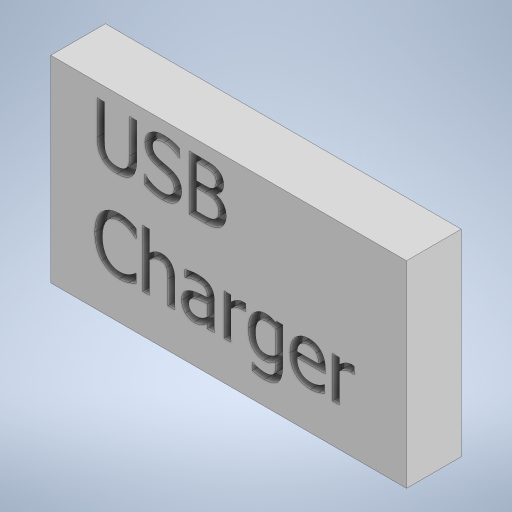
# Autodesk Inventor part: rapoukUSBChargerv0
Saved by Autodesk Inventor 2024 (Build 280153000, 153)
## iProperties
Created: 2024-02-03
Part Number: rapoukUSBChargerv0
Material: Všeobecné
Document SubType Name: Modeling
Designer: Roman Suk
Density: 1 g/cm^3
Appearance: Výchozí
Author: Roman Suk
MASSSFP: 400 g
SFP: 4HR
Autodesk Inventor part; units mm, degrees
ref_plane "YZ Plane" through (0, 0, 0) normal (1, 0, 0) x (0, 1, 0)
ref_plane "XZ Plane" through (0, 0, 0) normal (0, 1, 0) x (-1, 0, 0)
ref_plane "XY Plane" through (0, 0, 0) normal (0, 0, 1) x (1, 0, 0)
sketch "Sketch2" plane through (0, 0, 0) normal (0, 0, 1) x (1, 0, 0)
  line L0 (-16.25, -9) -> (16.25, -9)
  line L1 (16.25, -9) -> (16.25, 9)
  line L2 (16.25, 9) -> (-16.25, 9)
  line L3 (-16.25, 9) -> (-16.25, -9)
  line L4 (-16.25, -9) -> (16.25, 9) construction
  line L5 (16.25, -9) -> (-16.25, 9) construction
  point P0 (0, 0)
  dimension "d2" = 32.5
  dimension "d3" = 18
  constraints: 12 end point, 2 midpoint, 2 parallel, 1 horizontal, 1 perpendicular
  measures "d2" distance of L2.end L1.end
  measures "d3" distance of L1.end L0.end
extrude "Extrusion2" add sketch "Sketch2" along normal blind 5
sketch "Sketch3" plane through (0, 0, 5) normal (0, 0, 1) x (1, 0, 0)
  line L0 (-12.4484, 7.8564) -> (20.0688, 7.8564) construction
  line L1 (20.0688, 7.8564) -> (20.0688, -10.2359) construction
  line L2 (20.0688, -10.2359) -> (-12.4484, -10.2359) construction
  line L3 (-12.4484, -10.2359) -> (-12.4484, 7.8564) construction
  spline S0 degree 2 poles (-10.1956, 2.662) (-10.6373, 2.662) (-11.2937, 2.8929) (-11.5246, 3.1239) knots 0 0 0 1 2 2 2
  spline S1 degree 2 poles (-11.5246, 3.1239) (-11.788, 3.3832) (-12.0027, 4.1125) (-12.0027, 4.6474) knots 0 0 0 1 2 2 2
  line L4 (-12.0027, 4.6474) -> (-12.0027, 7.7673)
  line L5 (-12.0027, 7.7673) -> (-11.3382, 7.7673)
  line L6 (-11.3382, 7.7673) -> (-11.3382, 4.6474)
  spline S2 degree 2 poles (-11.3382, 4.6474) (-11.3382, 4.2989) (-11.2491, 3.8289) (-11.1235, 3.6385) knots 0 0 0 1 2 2 2
  spline S3 degree 2 poles (-11.1235, 3.6385) (-10.9898, 3.4359) (-10.5279, 3.2292) (-10.1956, 3.2292) knots 0 0 0 1 2 2 2
  spline S4 degree 2 poles (-10.1956, 3.2292) (-9.8836, 3.2292) (-9.3974, 3.4359) (-9.2637, 3.6385) knots 0 0 0 1 2 2 2
  spline S5 degree 2 poles (-9.2637, 3.6385) (-9.1381, 3.8289) (-9.0489, 4.2949) (-9.0489, 4.6312) knots 0 0 0 1 2 2 2
  line L7 (-9.0489, 4.6312) -> (-9.0489, 7.7673)
  line L8 (-9.0489, 7.7673) -> (-8.3844, 7.7673)
  line L9 (-8.3844, 7.7673) -> (-8.3844, 4.6474)
  spline S6 degree 2 poles (-8.3844, 4.6474) (-8.3844, 4.1247) (-8.5951, 3.3791) (-8.8625, 3.1239) knots 0 0 0 1 2 2 2
  spline S7 degree 2 poles (-8.8625, 3.1239) (-9.1016, 2.8889) (-9.7337, 2.662) (-10.1956, 2.662) knots 0 0 0 1 2 2 2
  spline S8 degree 2 poles (-6.0384, 2.6782) (-6.5813, 2.6782) (-7.3431, 2.9051) (-7.6794, 3.0671) knots 0 0 0 1 2 2 2
  line L10 (-7.6794, 3.0671) -> (-7.6794, 3.9018)
  line L11 (-7.6794, 3.9018) -> (-7.6308, 3.9018)
  spline S9 degree 2 poles (-7.6308, 3.9018) (-7.3026, 3.5939) (-6.4719, 3.2535) (-6.087, 3.2535) knots 0 0 0 1 2 2 2
  spline S10 degree 2 poles (-6.087, 3.2535) (-5.536, 3.2535) (-4.9727, 3.7114) (-4.9727, 4.0882) knots 0 0 0 1 2 2 2
  spline S11 degree 2 poles (-4.9727, 4.0882) (-4.9727, 4.388) (-5.2685, 4.7608) (-5.5886, 4.854) knots 0 0 0 1 2 2 2
  spline S12 degree 2 poles (-5.5886, 4.854) (-5.8196, 4.9188) (-6.2045, 5.008) (-6.4922, 5.0809) knots 0 0 0 1 2 2 2
  spline S13 degree 2 poles (-6.4922, 5.0809) (-6.7515, 5.1498) (-7.1608, 5.3564) (-7.3188, 5.5226) knots 0 0 0 1 2 2 2
  spline S14 degree 2 poles (-7.3188, 5.5226) (-7.4727, 5.6887) (-7.6429, 6.1344) (-7.6429, 6.4261) knots 0 0 0 1 2 2 2
  spline S15 degree 2 poles (-7.6429, 6.4261) (-7.6429, 7.0339) (-6.6948, 7.8564) (-5.9614, 7.8564) knots 0 0 0 1 2 2 2
  spline S16 degree 2 poles (-5.9614, 7.8564) (-5.54, 7.8564) (-4.7945, 7.6903) (-4.4744, 7.5323) knots 0 0 0 1 2 2 2
  line L12 (-4.4744, 7.5323) -> (-4.4744, 6.7381)
  line L13 (-4.4744, 6.7381) -> (-4.523, 6.7381)
  spline S17 degree 2 poles (-4.523, 6.7381) (-4.762, 6.9569) (-5.5076, 7.2811) (-5.9168, 7.2811) knots 0 0 0 1 2 2 2
  spline S18 degree 2 poles (-5.9168, 7.2811) (-6.3787, 7.2811) (-6.9501, 6.8475) (-6.9501, 6.495) knots 0 0 0 1 2 2 2
  spline S19 degree 2 poles (-6.9501, 6.495) (-6.9501, 6.179) (-6.6138, 5.8021) (-6.2977, 5.7171) knots 0 0 0 1 2 2 2
  spline S20 degree 2 poles (-6.2977, 5.7171) (-6.087, 5.6603) (-5.4752, 5.5145) (-5.2726, 5.4537) knots 0 0 0 1 2 2 2
  spline S21 degree 2 poles (-5.2726, 5.4537) (-4.758, 5.2957) (-4.2799, 4.6595) (-4.2799, 4.1936) knots 0 0 0 1 2 2 2
  spline S22 degree 2 poles (-4.2799, 4.1936) (-4.2799, 3.8978) (-4.5189, 3.3305) (-4.7337, 3.132) knots 0 0 0 1 2 2 2
  spline S23 degree 2 poles (-4.7337, 3.132) (-4.9727, 2.9132) (-5.5805, 2.6782) (-6.0384, 2.6782) knots 0 0 0 1 2 2 2
  spline S24 degree 2 poles (-0.2118, 4.303) (-0.2118, 3.9302) (-0.4954, 3.3589) (-0.7304, 3.1725) knots 0 0 0 1 2 2 2
  spline S25 degree 2 poles (-0.7304, 3.1725) (-1.0141, 2.9537) (-1.6583, 2.7673) (-2.1689, 2.7673) knots 0 0 0 1 2 2 2
  line L14 (-2.1689, 2.7673) -> (-3.6032, 2.7673)
  line L15 (-3.6032, 2.7673) -> (-3.6032, 7.7673)
  line L16 (-3.6032, 7.7673) -> (-2.2783, 7.7673)
  spline S26 degree 2 poles (-2.2783, 7.7673) (-1.7434, 7.7673) (-1.2086, 7.6984) (-0.9655, 7.5647) knots 0 0 0 1 2 2 2
  spline S27 degree 2 poles (-0.9655, 7.5647) (-0.694, 7.4229) (-0.4468, 6.9569) (-0.4468, 6.6409) knots 0 0 0 1 2 2 2
  spline S28 degree 2 poles (-0.4468, 6.6409) (-0.4468, 6.2884) (-0.8196, 5.7292) (-1.1478, 5.5712) knots 0 0 0 1 2 2 2
  line L17 (-1.1478, 5.5712) -> (-1.1478, 5.5469)
  spline S29 degree 2 poles (-1.1478, 5.5469) (-0.7021, 5.4253) (-0.2118, 4.7811) (-0.2118, 4.303) knots 0 0 0 1 2 2 2
  spline S30 degree 2 poles (-0.9047, 4.2746) (-0.9047, 4.5582) (-1.0667, 4.9229) (-1.3099, 5.0526) knots 0 0 0 1 2 2 2
  spline S31 degree 2 poles (-1.3099, 5.0526) (-1.4679, 5.1336) (-1.8407, 5.1822) (-2.1851, 5.1822) knots 0 0 0 1 2 2 2
  line L18 (-2.1851, 5.1822) -> (-2.9387, 5.1822)
  line L19 (-2.9387, 5.1822) -> (-2.9387, 3.3346)
  line L20 (-2.9387, 3.3346) -> (-2.3998, 3.3346)
  spline S32 degree 2 poles (-2.3998, 3.3346) (-1.9622, 3.3346) (-1.4598, 3.4156) (-1.2653, 3.5453) knots 0 0 0 1 2 2 2
  spline S33 degree 2 poles (-1.2653, 3.5453) (-1.0789, 3.679) (-0.9047, 4.0112) (-0.9047, 4.2746) knots 0 0 0 1 2 2 2
  spline S34 degree 2 poles (-1.1397, 6.5477) (-1.1397, 6.726) (-1.2612, 6.9934) (-1.395, 7.0704) knots 0 0 0 1 2 2 2
  spline S35 degree 2 poles (-1.395, 7.0704) (-1.557, 7.1595) (-1.9501, 7.2) (-2.3026, 7.2) knots 0 0 0 1 2 2 2
  line L21 (-2.3026, 7.2) -> (-2.9387, 7.2)
  line L22 (-2.9387, 7.2) -> (-2.9387, 5.7373)
  line L23 (-2.9387, 5.7373) -> (-2.1851, 5.7373)
  spline S36 degree 2 poles (-2.1851, 5.7373) (-1.8731, 5.7373) (-1.5773, 5.8021) (-1.4193, 5.9034) knots 0 0 0 1 2 2 2
  spline S37 degree 2 poles (-1.4193, 5.9034) (-1.2653, 6.0007) (-1.1397, 6.3127) (-1.1397, 6.5477) knots 0 0 0 1 2 2 2
  spline S38 degree 2 poles (-9.989, -5.5542) (-10.4752, -5.5542) (-11.2977, -5.226) (-11.5975, -4.8978) knots 0 0 0 1 2 2 2
  spline S39 degree 2 poles (-11.5975, -4.8978) (-11.8974, -4.5737) (-12.2256, -3.6012) (-12.2256, -2.9691) knots 0 0 0 1 2 2 2
  spline S40 degree 2 poles (-12.2256, -2.9691) (-12.2256, -2.3411) (-11.9055, -1.4092) (-11.6016, -1.0647) knots 0 0 0 1 2 2 2
  spline S41 degree 2 poles (-11.6016, -1.0647) (-11.3018, -0.7284) (-10.4833, -0.3759) (-9.9768, -0.3759) knots 0 0 0 1 2 2 2
  spline S42 degree 2 poles (-9.9768, -0.3759) (-9.7256, -0.3759) (-9.2839, -0.4489) (-9.0975, -0.5056) knots 0 0 0 1 2 2 2
  spline S43 degree 2 poles (-9.0975, -0.5056) (-8.9355, -0.5583) (-8.5992, -0.7082) (-8.433, -0.7973) knots 0 0 0 1 2 2 2
  line L24 (-8.433, -0.7973) -> (-8.433, -1.5996)
  line L25 (-8.433, -1.5996) -> (-8.4857, -1.5996)
  spline S44 degree 2 poles (-8.4857, -1.5996) (-8.5749, -1.5186) (-8.8504, -1.2916) (-9.0489, -1.1822) knots 0 0 0 1 2 2 2
  spline S45 degree 2 poles (-9.0489, -1.1822) (-9.2394, -1.0769) (-9.6891, -0.9432) (-9.9808, -0.9432) knots 0 0 0 1 2 2 2
  spline S46 degree 2 poles (-9.9808, -0.9432) (-10.3009, -0.9432) (-10.8723, -1.2066) (-11.087, -1.4578) knots 0 0 0 1 2 2 2
  spline S47 degree 2 poles (-11.087, -1.4578) (-11.2977, -1.713) (-11.5327, -2.4869) (-11.5327, -2.9691) knots 0 0 0 1 2 2 2
  spline S48 degree 2 poles (-11.5327, -2.9691) (-11.5327, -3.4837) (-11.2856, -4.2252) (-11.0708, -4.4805) knots 0 0 0 1 2 2 2
  spline S49 degree 2 poles (-11.0708, -4.4805) (-10.8601, -4.7276) (-10.2969, -4.9788) (-9.9808, -4.9788) knots 0 0 0 1 2 2 2
  spline S50 degree 2 poles (-9.9808, -4.9788) (-9.6932, -4.9788) (-9.2029, -4.837) (-9.0125, -4.7317) knots 0 0 0 1 2 2 2
  spline S51 degree 2 poles (-9.0125, -4.7317) (-8.8301, -4.6263) (-8.5586, -4.4075) (-8.4817, -4.3305) knots 0 0 0 1 2 2 2
  line L26 (-8.4817, -4.3305) -> (-8.433, -4.3305)
  line L27 (-8.433, -4.3305) -> (-8.433, -5.1247)
  spline S52 degree 2 poles (-8.433, -5.1247) (-8.5992, -5.2017) (-8.8909, -5.3435) (-9.0975, -5.4083) knots 0 0 0 1 2 2 2
  spline S53 degree 2 poles (-9.0975, -5.4083) (-9.3163, -5.4813) (-9.6891, -5.5542) (-9.989, -5.5542) knots 0 0 0 1 2 2 2
  line L28 (-4.916, -5.4651) -> (-5.5481, -5.4651)
  line L29 (-5.5481, -5.4651) -> (-5.5481, -3.3257)
  spline S54 degree 2 poles (-5.5481, -3.3257) (-5.5481, -3.0664) (-5.5967, -2.6207) (-5.6697, -2.4869) knots 0 0 0 1 2 2 2
  spline S55 degree 2 poles (-5.6697, -2.4869) (-5.7467, -2.3451) (-6.0222, -2.2074) (-6.2572, -2.2074) knots 0 0 0 1 2 2 2
  spline S56 degree 2 poles (-6.2572, -2.2074) (-6.4922, -2.2074) (-6.9906, -2.4586) (-7.2296, -2.6612) knots 0 0 0 1 2 2 2
  line L30 (-7.2296, -2.6612) -> (-7.2296, -5.4651)
  line L31 (-7.2296, -5.4651) -> (-7.8617, -5.4651)
  line L32 (-7.8617, -5.4651) -> (-7.8617, -0.2422)
  line L33 (-7.8617, -0.2422) -> (-7.2296, -0.2422)
  line L34 (-7.2296, -0.2422) -> (-7.2296, -2.1304)
  spline S57 degree 2 poles (-7.2296, -2.1304) (-6.946, -1.8751) (-6.399, -1.6077) (-6.0911, -1.6077) knots 0 0 0 1 2 2 2
  spline S58 degree 2 poles (-6.0911, -1.6077) (-5.54, -1.6077) (-4.916, -2.337) (-4.916, -3.0299) knots 0 0 0 1 2 2 2
  line L35 (-4.916, -3.0299) -> (-4.916, -5.4651)
  spline S59 degree 2 poles (-1.9379, -5.068) (-2.0149, -5.1247) (-2.2742, -5.3273) (-2.3958, -5.3881) knots 0 0 0 1 2 2 2
  spline S60 degree 2 poles (-2.3958, -5.3881) (-2.5619, -5.4772) (-2.8739, -5.5704) (-3.1575, -5.5704) knots 0 0 0 1 2 2 2
  spline S61 degree 2 poles (-3.1575, -5.5704) (-3.3885, -5.5704) (-3.8058, -5.3962) (-3.9638, -5.2382) knots 0 0 0 1 2 2 2
  spline S62 degree 2 poles (-3.9638, -5.2382) (-4.1138, -5.0842) (-4.2961, -4.6304) (-4.2961, -4.3792) knots 0 0 0 1 2 2 2
  spline S63 degree 2 poles (-4.2961, -4.3792) (-4.2961, -3.9902) (-3.9679, -3.4391) (-3.6113, -3.2811) knots 0 0 0 1 2 2 2
  spline S64 degree 2 poles (-3.6113, -3.2811) (-3.2953, -3.1352) (-2.4363, -3.0258) (-1.9379, -2.9975) knots 0 0 0 1 2 2 2
  line L36 (-1.9379, -2.9975) -> (-1.9379, -2.8759)
  spline S65 degree 2 poles (-1.9379, -2.8759) (-1.9379, -2.6571) (-2.0716, -2.3856) (-2.1932, -2.3087) knots 0 0 0 1 2 2 2
  spline S66 degree 2 poles (-2.1932, -2.3087) (-2.3147, -2.2317) (-2.6632, -2.1831) (-2.8496, -2.1831) knots 0 0 0 1 2 2 2
  spline S67 degree 2 poles (-2.8496, -2.1831) (-3.0684, -2.1831) (-3.6599, -2.3127) (-3.9557, -2.4383) knots 0 0 0 1 2 2 2
  line L37 (-3.9557, -2.4383) -> (-3.9922, -2.4383)
  line L38 (-3.9922, -2.4383) -> (-3.9922, -1.7941)
  spline S68 degree 2 poles (-3.9922, -1.7941) (-3.818, -1.7455) (-3.1656, -1.6239) (-2.8455, -1.6239) knots 0 0 0 1 2 2 2
  spline S69 degree 2 poles (-2.8455, -1.6239) (-2.4565, -1.6239) (-1.9257, -1.7455) (-1.715, -1.9035) knots 0 0 0 1 2 2 2
  spline S70 degree 2 poles (-1.715, -1.9035) (-1.5084, -2.0574) (-1.3058, -2.5477) (-1.3058, -2.9002) knots 0 0 0 1 2 2 2
  line L39 (-1.3058, -2.9002) -> (-1.3058, -5.4651)
  line L40 (-1.3058, -5.4651) -> (-1.9379, -5.4651)
  line L41 (-1.9379, -5.4651) -> (-1.9379, -5.068)
  line L42 (-1.9379, -4.5412) -> (-1.9379, -3.4999)
  spline S71 degree 2 poles (-1.9379, -3.4999) (-2.1648, -3.5202) (-2.8496, -3.5891) (-3.0643, -3.6539) knots 0 0 0 1 2 2 2
  spline S72 degree 2 poles (-3.0643, -3.6539) (-3.3155, -3.7309) (-3.6437, -4.051) (-3.6437, -4.3346) knots 0 0 0 1 2 2 2
  spline S73 degree 2 poles (-3.6437, -4.3346) (-3.6437, -4.6587) (-3.2791, -4.9869) (-2.9306, -4.9869) knots 0 0 0 1 2 2 2
  spline S74 degree 2 poles (-2.9306, -4.9869) (-2.6348, -4.9869) (-2.1486, -4.7317) (-1.9379, -4.5412) knots 0 0 0 1 2 2 2
  line L43 (1.571, -2.3897) -> (1.5386, -2.3897)
  spline S75 degree 2 poles (1.5386, -2.3897) (1.4657, -2.3694) (1.3076, -2.3613) (1.1982, -2.3613) knots 0 0 0 1 2 2 2
  spline S76 degree 2 poles (1.1982, -2.3613) (0.943, -2.3613) (0.4405, -2.5842) (0.2136, -2.803) knots 0 0 0 1 2 2 2
  line L44 (0.2136, -2.803) -> (0.2136, -5.4651)
  line L45 (0.2136, -5.4651) -> (-0.4185, -5.4651)
  line L46 (-0.4185, -5.4651) -> (-0.4185, -1.713)
  line L47 (-0.4185, -1.713) -> (0.2136, -1.713)
  line L48 (0.2136, -1.713) -> (0.2136, -2.2722)
  spline S77 degree 2 poles (0.2136, -2.2722) (0.558, -1.9643) (1.0726, -1.713) (1.3157, -1.713) knots 0 0 0 1 2 2 2
  spline S78 degree 2 poles (1.3157, -1.713) (1.413, -1.713) (1.5102, -1.7211) (1.571, -1.7333) knots 0 0 0 1 2 2 2
  line L49 (1.571, -1.7333) -> (1.571, -2.3897)
  spline S79 degree 2 poles (2.195, -6.0647) (2.2598, -6.0931) (2.507, -6.1822) (2.665, -6.2187) knots 0 0 0 1 2 2 2
  spline S80 degree 2 poles (2.665, -6.2187) (2.8392, -6.2633) (3.135, -6.316) (3.3093, -6.316) knots 0 0 0 1 2 2 2
  spline S81 degree 2 poles (3.3093, -6.316) (3.601, -6.316) (4.0062, -6.162) (4.1196, -6.0242) knots 0 0 0 1 2 2 2
  spline S82 degree 2 poles (4.1196, -6.0242) (4.229, -5.8865) (4.3141, -5.5258) (4.3141, -5.2949) knots 0 0 0 1 2 2 2
  line L50 (4.3141, -5.2949) -> (4.3141, -4.9667)
  spline S83 degree 2 poles (4.3141, -4.9667) (4.0589, -5.1895) (3.5686, -5.4002) (3.1999, -5.4002) knots 0 0 0 1 2 2 2
  spline S84 degree 2 poles (3.1999, -5.4002) (2.5597, -5.4002) (1.802, -4.448) (1.802, -3.5526) knots 0 0 0 1 2 2 2
  spline S85 degree 2 poles (1.802, -3.5526) (1.802, -3.0866) (2.0653, -2.3654) (2.2841, -2.1101) knots 0 0 0 1 2 2 2
  spline S86 degree 2 poles (2.2841, -2.1101) (2.4948, -1.8711) (3.0743, -1.6077) (3.3822, -1.6077) knots 0 0 0 1 2 2 2
  spline S87 degree 2 poles (3.3822, -1.6077) (3.6739, -1.6077) (4.0994, -1.7455) (4.3141, -1.8711) knots 0 0 0 1 2 2 2
  line L51 (4.3141, -1.8711) -> (4.3506, -1.713)
  line L52 (4.3506, -1.713) -> (4.9462, -1.713)
  line L53 (4.9462, -1.713) -> (4.9462, -5.0356)
  spline S88 degree 2 poles (4.9462, -5.0356) (4.9462, -5.9918) (4.1156, -6.8832) (3.2606, -6.8832) knots 0 0 0 1 2 2 2
  spline S89 degree 2 poles (3.2606, -6.8832) (2.9851, -6.8832) (2.4097, -6.7941) (2.1626, -6.7211) knots 0 0 0 1 2 2 2
  line L54 (2.1626, -6.7211) -> (2.1626, -6.0647)
  line L55 (2.1626, -6.0647) -> (2.195, -6.0647)
  line L56 (4.3141, -4.448) -> (4.3141, -2.3856)
  spline S90 degree 2 poles (4.3141, -2.3856) (4.0791, -2.2722) (3.682, -2.175) (3.4835, -2.175) knots 0 0 0 1 2 2 2
  spline S91 degree 2 poles (3.4835, -2.175) (3.0054, -2.175) (2.4543, -2.88) (2.4543, -3.5404) knots 0 0 0 1 2 2 2
  spline S92 degree 2 poles (2.4543, -3.5404) (2.4543, -4.1644) (2.8717, -4.8168) (3.3417, -4.8168) knots 0 0 0 1 2 2 2
  spline S93 degree 2 poles (3.3417, -4.8168) (3.5888, -4.8168) (4.1075, -4.6223) (4.3141, -4.448) knots 0 0 0 1 2 2 2
  spline S94 degree 2 poles (7.4908, -5.5502) (6.5913, -5.5502) (5.6026, -4.5412) (5.6026, -3.6093) knots 0 0 0 1 2 2 2
  spline S95 degree 2 poles (5.6026, -3.6093) (5.6026, -2.6936) (6.5629, -1.6077) (7.3368, -1.6077) knots 0 0 0 1 2 2 2
  spline S96 degree 2 poles (7.3368, -1.6077) (7.6853, -1.6077) (8.2242, -1.8103) (8.4227, -2.025) knots 0 0 0 1 2 2 2
  spline S97 degree 2 poles (8.4227, -2.025) (8.6253, -2.2398) (8.8401, -2.8597) (8.8401, -3.3095) knots 0 0 0 1 2 2 2
  line L57 (8.8401, -3.3095) -> (8.8401, -3.6539)
  line L58 (8.8401, -3.6539) -> (6.2428, -3.6539)
  spline S98 degree 2 poles (6.2428, -3.6539) (6.2428, -4.3062) (6.8992, -4.9991) (7.4827, -4.9991) knots 0 0 0 1 2 2 2
  spline S99 degree 2 poles (7.4827, -4.9991) (7.6893, -4.9991) (8.0905, -4.9059) (8.2525, -4.833) knots 0 0 0 1 2 2 2
  spline S100 degree 2 poles (8.2525, -4.833) (8.4227, -4.7519) (8.6577, -4.6101) (8.7347, -4.5453) knots 0 0 0 1 2 2 2
  line L59 (8.7347, -4.5453) -> (8.7712, -4.5453)
  line L60 (8.7712, -4.5453) -> (8.7712, -5.2341)
  spline S101 degree 2 poles (8.7712, -5.2341) (8.6618, -5.2787) (8.3295, -5.4083) (8.1999, -5.4448) knots 0 0 0 1 2 2 2
  spline S102 degree 2 poles (8.1999, -5.4448) (8.0175, -5.4975) (7.7177, -5.5502) (7.4908, -5.5502) knots 0 0 0 1 2 2 2
  spline S103 degree 2 poles (8.2242, -3.1717) (8.2161, -2.9164) (8.1107, -2.5437) (8.0094, -2.4181) knots 0 0 0 1 2 2 2
  spline S104 degree 2 poles (8.0094, -2.4181) (7.9, -2.2762) (7.5556, -2.1263) (7.3003, -2.1263) knots 0 0 0 1 2 2 2
  spline S105 degree 2 poles (7.3003, -2.1263) (7.0491, -2.1263) (6.6966, -2.2762) (6.5508, -2.4221) knots 0 0 0 1 2 2 2
  spline S106 degree 2 poles (6.5508, -2.4221) (6.4089, -2.572) (6.2631, -2.9327) (6.2428, -3.1717) knots 0 0 0 1 2 2 2
  line L61 (6.2428, -3.1717) -> (8.2242, -3.1717)
  line L62 (11.4697, -2.3897) -> (11.4373, -2.3897)
  spline S107 degree 2 poles (11.4373, -2.3897) (11.3644, -2.3694) (11.2063, -2.3613) (11.0969, -2.3613) knots 0 0 0 1 2 2 2
  spline S108 degree 2 poles (11.0969, -2.3613) (10.8417, -2.3613) (10.3392, -2.5842) (10.1123, -2.803) knots 0 0 0 1 2 2 2
  line L63 (10.1123, -2.803) -> (10.1123, -5.4651)
  line L64 (10.1123, -5.4651) -> (9.4803, -5.4651)
  line L65 (9.4803, -5.4651) -> (9.4803, -1.713)
  line L66 (9.4803, -1.713) -> (10.1123, -1.713)
  line L67 (10.1123, -1.713) -> (10.1123, -2.2722)
  spline S109 degree 2 poles (10.1123, -2.2722) (10.4568, -1.9643) (10.9713, -1.713) (11.2144, -1.713) knots 0 0 0 1 2 2 2
  spline S110 degree 2 poles (11.2144, -1.713) (11.3117, -1.713) (11.4089, -1.7211) (11.4697, -1.7333) knots 0 0 0 1 2 2 2
  line L68 (11.4697, -1.7333) -> (11.4697, -2.3897)
  point P0 (0, 0)
  constraints: 2 other
extrude "Extrusion3" cut sketch "Sketch3" against normal blind 1
body "Solid2"
